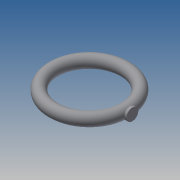
# Autodesk Inventor part: ringCentering
Saved by Autodesk Inventor 2014 SP1 (Build 180222100, 222)
## iProperties
Created: 2014-08-29
Part Number: ringCentering
Material: Generic
Document SubType Name: Modeling
Designer: Dave
Density: 1 g/cm^3
Appearance: Default
Author: Dave
Autodesk Inventor part; units mm, degrees
ref_plane "XZ Plane" through (0, 0, 0) normal (0, 1, 0) x (-1, 0, 0)
ref_plane "XY Plane" through (0, 0, 0) normal (0, 0, 1) x (1, 0, 0)
sketch "Sketch1" plane through (0, 0, 0) normal (0, 0, 1) x (1, 0, 0)
  circle A0 centre (0, 0) radius 3.175
  line L0 (-19.05, 7.7404) -> (-19.05, -6.3643) construction
  dimension "d0" = 6.35
  dimension "d1" = 19.05
  constraints: 2 end point, 1 centre point, 1 coincident, 1 vertical
  measures "d0" diameter of A0
  measures "d1" distance from line of A0.centre L0
revolve "Revolution1" add sketch "Sketch1" angle 360 about axis through (-19.05, 7.7404, 0) along (0, -1, 0)
ref_plane "Work Plane1" through (2.54, 0, 0) normal (1, 0, 0) x (0, 1, 0)
sketch "Sketch2" plane through (2.54, 0, 0) normal (1, 0, 0) x (0, 1, 0)
  circle A0 centre (0, 0) radius 3.175
  dimension "d4" = 6.35
  constraints: 1 centre point, 1 coincident
  measures "d4" diameter of A0
extrude "Extrusion1" add sketch "Sketch2" along normal blind 1.27
body "Solid1"
